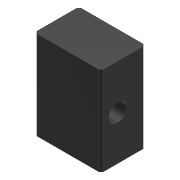
# Autodesk Inventor part: 10-006-ACTR-FIX
Saved by Autodesk Inventor 2018 (Build 220112000, 112)
## iProperties
Created: 2017-07-31
Part Number: 10-006-ACTR-FIX
Material: Steel
Document SubType Name: Modeling
Designer: feesmrt
Density: 7.85 g/cm^3
Appearance: Smooth - Black
Author: feesmrt
Autodesk Inventor part; units mm, degrees
ref_plane "YZ Plane" through (0, 0, 0) normal (1, 0, 0) x (0, 1, 0)
ref_plane "XZ Plane" through (0, 0, 0) normal (0, 1, 0) x (-1, 0, 0)
ref_plane "XY Plane" through (0, 0, 0) normal (0, 0, 1) x (1, 0, 0)
sketch "Sketch1" plane through (0, 0, 0) normal (1, 0, 0) x (0, 1, 0)
  line L0 (-20, 40) -> (20, 40)
  line L1 (20, 40) -> (20, -40)
  line L2 (20, -40) -> (-20, -40)
  line L3 (-20, -40) -> (-20, 40)
  line L4 (-20, 40) -> (20, -40) construction
  line L5 (20, 40) -> (-20, -40) construction
  circle A0 centre (-5, 0) radius 8
  line L6 (0, 56) -> (0, -56) construction
  line L7 (-28, 0) -> (28, 0) construction
  point P0 (0, 0)
  dimension "d0" = 80
  dimension "d1" = 40
  dimension "d2" = 15
  dimension "d3" = 16
  constraints: 12 end point, 2 midpoint, 2 parallel, 1 centre point, 1 horizontal, 1 perpendicular, 1 point on line
  measures "d0" distance of L0.end L1.end
  measures "d1" distance of L1.end L2.end
  measures "d2" distance from line of L3 A0.centre
  measures "d3" diameter of A0
extrude "Extrusion1" add sketch "Sketch1" along normal mid plane 60
chamfer "Chamfer1" distance 2 angle 45 4 edges at (-30, -20, 0) (-30, 20, 0) (30, 20, 0) (30, -20, 0)
body "Solid1"
